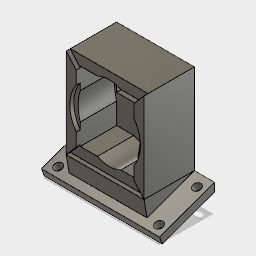
CameraMount v4 (Autodesk Fusion 360 design; units mm, degrees)
Autodesk Fusion 360 part; units mm, degrees
sketch "Sketch1" plane through (0, 0, 0) normal (0, 1, 0) x (1, 0, 0)
  line L0 (43.18, 7.62) -> (-5.842, 7.62)
  line L1 (-5.842, 7.62) -> (-5.842, -21.59)
  line L2 (-5.842, -21.59) -> (43.18, -21.59)
  line L3 (43.18, -21.59) -> (43.18, 7.62)
  dimension "d9" = 49.022
  dimension "d10" = 29.21
  constraint horizontal L0
  constraint vertical L1
  constraint horizontal L2
  constraint vertical L3
extrude "Extrude1" add sketch "Sketch1" along normal blind 56.515 makes body 1
sketch "Sketch2" plane through (0, 0, 21.59) normal (0, 0, 1) x (1, 0, 0)
  line L0 (-5.842, 0) -> (43.18, 0)
  line L1 (43.18, 0) -> (43.18, 56.515)
  line L2 (43.18, 56.515) -> (-5.842, 56.515)
  line L3 (-5.842, 56.515) -> (-5.842, 0)
  line L4 (0.508, 50.165) -> (36.83, 50.165)
  line L5 (36.83, 50.165) -> (36.83, 6.35)
  line L6 (36.83, 6.35) -> (0.508, 6.35)
  line L7 (0.508, 6.35) -> (0.508, 50.165)
  dimension "d3" = 43.815
  dimension "d4" = 36.322
  dimension "d7" = 6.35
  dimension "d8" = 6.35
  constraint horizontal L4
  constraint vertical L5
  constraint horizontal L6
  constraint vertical L7
  measures "d3" distance of origin
  measures "d7" distance of L3 L7
  measures "d8" distance of L2 L4
extrude "Extrude2" cut sketch "Sketch2" against normal blind 22.86 contours L4 L5 L6 L7 bodies 1
sketch "Sketch3" plane through (0, 0, -1.27) normal (0, 0, 1) x (1, 0, 0)
  line L0 (0.508, 6.35) -> (36.83, 6.35)
  line L1 (36.83, 6.35) -> (36.83, 50.165)
  line L2 (36.83, 50.165) -> (0.508, 50.165)
  line L3 (0.508, 50.165) -> (0.508, 6.35)
  line L4 (36.83, 32.0675) -> (0, 32.0675)
  line L5 (0, 32.0675) -> (0, 24.4475)
  line L6 (0, 24.4475) -> (36.83, 24.4475)
  line L7 (36.83, 24.4475) -> (36.83, 32.0675)
  line L8 (-5.842, 0) -> (43.18, 0)
  line L9 (-5.842, 56.515) -> (43.18, 56.515)
  dimension "d11" = 7.62
  dimension "d12" = 24.4475
  dimension "d13" = 24.4475
  constraint horizontal L4
  constraint vertical L5
  constraint horizontal L6
  constraint vertical L7
  constraint coincident L1 origin
  measures "d11" distance of L4 L6
  measures "d12" distance of L6 L8
  measures "d13" distance of L4 L9
extrude "Extrude3" cut sketch "Sketch3" against normal blind 33.02 contours L1 L3 L4 L6 L7 bodies 1
sketch "Sketch4" plane through (0, 0, 21.59) normal (0, 0, 1) x (1, 0, 0)
  line L0 (36.83, 50.165) -> (36.83, 6.35)
  line L1 (36.83, 6.35) -> (0.508, 6.35)
  line L2 (0.508, 6.35) -> (0.508, 50.165)
  line L3 (0.508, 50.165) -> (36.83, 50.165)
  line L4 (-5.842, 0) -> (43.18, 0)
  line L5 (43.18, 0) -> (43.18, 56.515)
  line L6 (43.18, 56.515) -> (-5.842, 56.515)
  line L7 (-5.842, 56.515) -> (-5.842, 0)
  line L8 (43.18, 0) -> (-5.842, 56.515)
  line L9 (43.18, 56.515) -> (-5.842, 0)
  circle A0 centre (18.669, 28.2575) radius 22.225
  circle A1 centre (18.669, 28.2575) radius 15.875
  dimension "d16" = 44.45
  dimension "d17" = 31.75
  constraint midpoint L9
  constraint concentric A0 A1
  measures "d16" diameter of A0
  measures "d17" diameter of A1
extrude "Extrude4" add sketch "Sketch4" along normal blind 2.54 contours L0 L5 L8 L9 A0 | L2 L7 L8 L9 A0 bodies 1
sketch "Sketch5" plane through (0, 0, 21.59) normal (0, 0, 1) x (1, 0, 0)
  line L0 (-5.842, 56.515) -> (0.508, 49.1944)
  line L1 (0.508, 49.1944) -> (0.508, 50.165)
  line L2 (0.508, 50.165) -> (36.83, 50.165)
  line L3 (36.83, 50.165) -> (36.83, 49.1944)
  line L4 (36.83, 49.1944) -> (43.18, 56.515)
  line L5 (43.18, 56.515) -> (-5.842, 56.515)
  line L6 (0.508, 50.165) -> (36.83, 6.35)
  line L7 (36.83, 6.35) -> (36.83, 50.165)
  line L8 (0.508, 6.35) -> (36.83, 50.165)
  ellipse E0 centre (18.669, 28.2575) end of major axis (18.669, 51.9239) minor radius 19.4749
  line L9 (18.669, 4.5911) -> (18.669, 51.9239)
  line L10 (38.1439, 28.2575) -> (-0.8059, 28.2575)
  constraint perpendicular L2 L9
  constraint coincident E0
extrude "Extrude5" cut sketch "Sketch5" against normal blind 22.86 contours L2 E0 L9 | L2 L6 E0 L9 | L6 E0 L10 | L7 E0 L10 | L7 L8 E0 L10 | L2 E0 L9 | L2 L8 E0 L9 | L6 L7 E0 L10 | L8 E0 L9 | L6 E0 L9 | L8 E0 L10 | L7 E0 L10 bodies 1
sketch "Sketch6" plane through (43.18, 0, 0) normal (1, 0, 0) x (0, 0, -1)
  line L0 (-21.59, 0) -> (7.62, 0)
  line L1 (7.62, 0) -> (7.62, 56.515)
  line L2 (7.62, 56.515) -> (-21.59, 56.515)
  line L3 (-21.59, 56.515) -> (-24.13, 56.515)
  line L4 (-24.13, 56.515) -> (-24.13, 0)
  line L5 (-24.13, 0) -> (-21.59, 0)
  line L6 (7.62, 0) -> (-24.13, 0)
  line L7 (-22.2752, -10.881) -> (7.62, 0)
  line L8 (-24.13, 0) -> (-22.2752, -10.881)
  dimension "d22" = 20
  measures "d22" angle of L6 L7
extrude "Extrude6" add sketch "Sketch6" against normal blind 49.022 separate body contours L0 L5 L6 L7 L8 makes body 2
sketch "Sketch7" plane through (0, -2.449, -0.8914) normal (0, -0.939693, -0.34202) x (-1, 0, 0)
  line L0 (-43.18, 7.1605) -> (-43.18, -24.6534)
  line L1 (-43.18, -24.6534) -> (5.842, -24.6534)
  line L2 (5.842, -24.6534) -> (5.842, 7.1605)
  line L3 (5.842, 7.1605) -> (-43.18, 7.1605)
  line L4 (-55.88, 7.1399) -> (18.542, 7.1399)
  line L5 (18.542, 7.1399) -> (18.542, -29.7334)
  line L6 (18.542, -29.7334) -> (-55.88, -29.7334)
  line L7 (-55.88, -29.7334) -> (-55.88, 7.1399)
  dimension "d25" = 12.7
  dimension "d26" = 12.7
  dimension "d28" = 5.08
  dimension "d29" = 52.1339
  constraint horizontal L4
  constraint vertical L5
  constraint horizontal L6
  constraint vertical L7
  measures "d25" distance of L0 L7
  measures "d26" distance of L2 L5
  measures "d28" distance of L1 L6
  measures "d29" distance of L4 L6
extrude "Extrude7" add sketch "Sketch7" along normal blind 5.08 contours L0 L1 L2 L4 | L0 L1 L2 L4 L5 L6 L7 bodies 2 1
sketch "Sketch8" plane through (0, -7.2227, -2.6288) normal (0, -0.939693, -0.34202) x (-1, 0, 0)
  line L0 (-55.88, -29.7334) -> (18.542, -29.7334)
  line L1 (18.542, -29.7334) -> (18.542, 7.1399)
  line L2 (18.542, 7.1399) -> (-55.88, 7.1399)
  line L3 (-55.88, 7.1399) -> (-55.88, -29.7334)
  dimension "d32" = 25.4
  dimension "d33" = 5.08
  dimension "d34" = 5.08
  dimension "d35" = 25.4
  dimension "d36" = 5.08
  dimension "d37" = 63.5
  dimension "d38" = 63.5
  measures "d33" distance of L0 origin
  measures "d34" distance of L0 origin
  measures "d35" distance of origin
  measures "d36" distance of L3 origin
  measures "d38" distance of origin
hole "Hole1" at (-12.7, -15.6546, 20.5378) at (-12.7, -6.9673, -3.3304) at (50.8, -6.9673, -3.3304) at (50.8, -15.6546, 20.5378) direction (0, 0.939693, 0.34202) diameter 5.08 depth 25.4 tip angle 118 bodies 2 1
sketch "Sketch9" plane through (-18.542, 0, 0) normal (-1, 0, 0) x (0, 0, 1)
  line L0 (27.0489, -12.6184) -> (-7.6007, -0.007)
  line L1 (-7.6007, -0.007) -> (-9.3382, -4.7807)
  line L2 (-9.3382, -4.7807) -> (25.3114, -17.3921)
  line L3 (25.3114, -17.3921) -> (27.0489, -12.6184)
  line L4 (-7.6007, -0.007) -> (-7.6007, -7.0418)
  line L5 (-7.6007, -7.0418) -> (-12.5938, -5.2245)
  line L6 (-12.5938, -5.2245) -> (-7.6007, -0.007)
  constraint vertical L4
  constraint perpendicular L1 L5
extrude "Extrude8" cut sketch "Sketch9" against normal blind 81.28 contours L1 L2 L4 bodies 2
